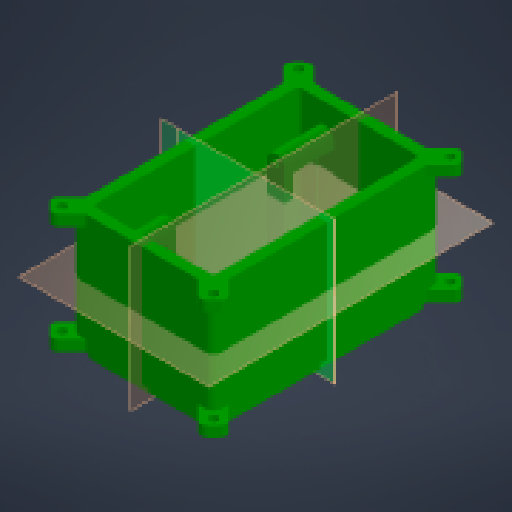
# Autodesk Inventor part: back_box_mid
Saved by Autodesk Inventor 2024 (Build 280153000, 153)
## iProperties
Created: 2023-05-15
Part Number: back_box_mid
Material: Типовые
Document SubType Name: Modeling
Designer: user
Density: 1 g/cm^3
Appearance: По умолчанию
Author: user
Autodesk Inventor part; units mm, degrees
sketch "Эскиз1" plane through (0, 0, 0) normal (0, 0, 1) x (1, 0, 0)
  line L0 (26.5, -50.5) -> (-26.5, -50.5) projected
  arc A0 (26.5, -50.5) -> (30.5, -46.5) centre (26.5, -46.5) ccw projected
  arc A1 (-30.5, -46.5) -> (-26.5, -50.5) centre (-26.5, -46.5) ccw projected
  line L1 (-30.5, -46.5) -> (-30.5, 46.5) projected
  line L2 (30.5, 46.5) -> (30.5, -46.5) projected
  arc A2 (30.5, 46.5) -> (26.5, 50.5) centre (26.5, 46.5) ccw projected
  line L3 (-26.5, 50.5) -> (26.5, 50.5) projected
  arc A3 (-26.5, 50.5) -> (-30.5, 46.5) centre (-26.5, 46.5) ccw projected
  line L4 (-26.5, -48.5) -> (26.5, -48.5)
  arc A4 (26.5, -48.5) -> (28.5, -46.5) centre (26.5, -46.5) ccw
  line L5 (28.5, -46.5) -> (28.5, 46.5)
  arc A5 (28.5, 46.5) -> (26.5, 48.5) centre (26.5, 46.5) ccw
  line L6 (26.5, 48.5) -> (-26.5, 48.5)
  arc A6 (-26.5, 48.5) -> (-28.5, 46.5) centre (-26.5, 46.5) ccw
  line L7 (-28.5, 46.5) -> (-28.5, -46.5)
  arc A7 (-28.5, -46.5) -> (-26.5, -48.5) centre (-26.5, -46.5) ccw
  point P0 (0, 0)
  dimension "d0" = 2
  constraints: 8 end point, 8 point on circle, 4 centre point, 7 other
  measures "d0" distance between parallel lines of L0 L4
extrude "Выдавливание1" add sketch "Эскиз1" against normal blind 5
sketch "Эскиз2" plane through (0, 0, 0) normal (0, 0, 1) x (1, 0, 0)
  line L0 (-29.5, -53.5) -> (29.5, -53.5) projected
  arc A0 (29.5, -53.5) -> (33.5, -49.5) centre (29.5, -49.5) ccw projected
  line L1 (33.5, -49.5) -> (33.5, 49.5) projected
  arc A1 (33.5, 49.5) -> (29.5, 53.5) centre (29.5, 49.5) ccw projected
  line L2 (29.5, 53.5) -> (-29.5, 53.5) projected
  arc A2 (-29.5, 53.5) -> (-33.5, 49.5) centre (-29.5, 49.5) ccw projected
  line L3 (-33.5, 49.5) -> (-33.5, -49.5) projected
  arc A3 (-33.5, -49.5) -> (-29.5, -53.5) centre (-29.5, -49.5) ccw projected
  line L4 (-28.5, -46.5) -> (-28.5, 46.5) projected
  arc A4 (-28.5, -46.5) -> (-26.5, -48.5) centre (-26.5, -46.5) ccw projected
  line L5 (26.5, -48.5) -> (-26.5, -48.5) projected
  arc A5 (26.5, -48.5) -> (28.5, -46.5) centre (26.5, -46.5) ccw projected
  line L6 (28.5, 46.5) -> (28.5, -46.5) projected
  arc A6 (28.5, 46.5) -> (26.5, 48.5) centre (26.5, 46.5) ccw projected
  line L7 (-26.5, 48.5) -> (26.5, 48.5) projected
  arc A7 (-26.5, 48.5) -> (-28.5, 46.5) centre (-26.5, 46.5) ccw projected
  point P0 (0, 0)
extrude "Выдавливание2" add sketch "Эскиз2" along normal blind 56
sketch "Эскиз3" plane through (-26.5, -48.5, -5) normal (0, 1, 0) x (1, 0, 0)
  circle A0 centre (10.4, -47.5) radius 1.6 projected
  circle A1 centre (10.4, -7.5) radius 1.6 projected
  line L0 (6.4, -7.5) -> (6.4, -47.5)
  line L1 (14.4, -47.5) -> (14.4, -7.5)
  arc A2 (6.4, -47.5) -> (14.4, -47.5) centre (10.4, -47.5) ccw
  arc A3 (14.4, -7.5) -> (6.4, -7.5) centre (10.4, -7.5) ccw
  point P0 (26.5, -5)
  dimension "d5" = 8
  constraints: 4 end point, 4 point on circle, 3 tangent, 2 centre point, 2 coincident, 1 parallel, 1 vertical
  measures "d5" distance between parallel lines of L0 L1
ref_plane "РабПлоскость1" through (-22.3, -25.5, -2.25) normal (0, -1, 0) x (1, 0, 0)
extrude "Выдавливание3" add sketch "Эскиз3" along normal up to surface (23 mm away)
shell "Оболочка1" thickness 4 removed faces 4 at (-20.087, -33.1667, 2.1781) at (-16.9001, -33.1667, 46.4192) at (-12.1, -40.8333, 29.1667) at (-20.1, -40.8333, 15.8333)
ref_plane "РабПлоскость2" through (-29.5, 0, 0) normal (0, 1, 0) x (1, 0, 0)
mirror "Зеркальное отражение1" about plane through (-29.5, 0, 0) normal (0, 1, 0) of "Выдавливание3"
shell "Оболочка2" thickness 4 removed faces 4 at (-15.2999, 33.1667, 46.4192) at (-20.087, 33.1667, 2.1781) at (-12.1, 40.8333, 29.1667) at (-20.1, 40.8333, 15.8333)
sketch "Эскиз5" plane through (0, 0, 0) normal (0, 0, -1) x (-1, 0, 0)
  circle A0 centre (35.6213, 55.6213) radius 2 projected
  line L0 (32.7929, 59.864) -> (26.4289, 53.5) projected
  line L1 (33.5, 46.4289) -> (39.864, 52.7929) projected
  line L2 (39.864, 57.0355) -> (37.0355, 59.864) projected
  arc A1 (37.0355, 59.864) -> (32.7929, 59.864) centre (34.9142, 57.7426) ccw projected
  arc A2 (39.864, 52.7929) -> (39.864, 57.0355) centre (37.7426, 54.9142) ccw projected
  arc A3 (33.5, 49.5) -> (29.5, 53.5) centre (29.5, 49.5) ccw projected
  line L3 (-29.5, 53.5) -> (29.5, 53.5) projected
  line L4 (26.4289, 53.5) -> (29.5, 53.5)
  line L5 (33.5, 49.5) -> (33.5, 46.4289)
  line L6 (33.5, 49.5) -> (33.5, -49.5) projected
  point P0 (0, 0)
  constraints: 4 end point, 2 point on line, 1 horizontal, 1 point on circle
extrude "Выдавливание4" add sketch "Эскиз5" against normal blind 5
ref_plane "РабПлоскость3" through (-29.5, 0, 56) normal (0, 1, 0) x (1, 0, 0)
ref_plane "РабПлоскость4" through (0, -49.5, 0) normal (1, 0, 0) x (0, 0, -1)
mirror "Зеркальное отражение2" about plane through (0, -49.5, 0) normal (1, 0, 0) of "Выдавливание4"
mirror "Зеркальное отражение3" about plane through (-29.5, 0, 56) normal (0, 1, 0) of "Выдавливание4", "Зеркальное отражение2"
ref_plane "РабПлоскость5" through (0, 0, 28) normal (0, 0, 1) x (1, 0, 0)
mirror "Зеркальное отражение4" about plane through (0, 0, 28) normal (0, 0, 1) of "Выдавливание4", "Зеркальное отражение2", "Зеркальное отражение3"
